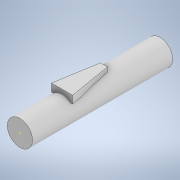
# Autodesk Inventor part: Part1
Saved by Autodesk Inventor 2021 (Build 250183000, 183)
## iProperties
Created: 2022-12-09
Part Number: Part1
Material: Generic
Document SubType Name: Modeling
Designer: user
Density: 1 g/cm^3
Appearance: Default
Author: user
Autodesk Inventor part; units mm, degrees
ref_plane "YZ Plane" through (0, 0, 0) normal (1, 0, 0) x (0, 1, 0)
ref_plane "XY Plane" through (0, 0, 0) normal (0, 0, 1) x (1, 0, 0)
sketch "Sketch4" plane through (0, 0, 0) normal (0, 0, 1) x (1, 0, 0)
  circle A0 centre (0, 0) radius 9
  dimension "d5" = 18
  constraints: 1 centre point, 1 coincident
  measures "d5" diameter of A0
sketch "Sketch5" plane through (0, 0, 0) normal (1, 0, 0) x (0, 1, 0)
  point P0 (0, 0)
ref_plane "Work Plane1" through (0, 9, 0) normal (0, 1, 0) x (-1, 0, 0)
sketch "Sketch6" plane through (0, 9, 0) normal (0, 1, 0) x (-1, 0, 0)
  line L0 (0, 0) -> (0, -100)
  line L1 (0, -30) -> (7.5, -30)
  line L2 (7.5, -30) -> (2.5456, -60)
  line L3 (2.5456, -60) -> (-2.4544, -60)
  line L4 (-2.4544, -60) -> (-7.5, -30)
  line L5 (-7.5, -30) -> (0, -30)
  dimension "d7" = 100
  dimension "d8" = 5
  dimension "d9" = 7.5
  dimension "d10" = 7.5
  dimension "d11" = 30
  dimension "d12" = 40
  constraints: 12 end point, 2 point on line, 1 collinear, 1 horizontal, 1 parallel, 1 vertical
  measures "d7" distance of L0.start L0.end
  measures "d8" distance of L2.end L3.end
  measures "d9" distance of L4.end L1.start
  measures "d10" distance of L1.start L1.end
  measures "d11" vertical distance of L2.end L1.end
  measures "d12" vertical distance of L3.end L0.end
extrude "Extrusion3" add sketch "Sketch4" against normal blind 100
extrude "Extrusion4" add sketch "Sketch6" along normal blind 3 and the other way blind 2.5
body "Solid3"
